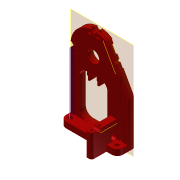
# Autodesk Inventor part: Cycl_marcoDerechoX
Saved by Autodesk Inventor 2015 SP2 (Build 190223200, 223)
## iProperties
Created: 2015-05-05
Material: Genérico
Document SubType Name: Modeling
Designer: E.Beroiz
Density: 1 g/cm^3
Appearance: Suave - Rojo
Description: Cycl_marcoDerechoX
Author: E.Beroiz
Autodesk Inventor part; units mm, degrees
ref_plane "YZ Plane" through (0, 0, 0) normal (1, 0, 0) x (0, 1, 0)
sketch "Boceto1" plane through (0, 0, 0) normal (0, 0, 1) x (1, 0, 0)
  line L0 (-49.75, 14.5) -> (49.75, 14.5)
  line L1 (49.75, 14.5) -> (49.75, -14.5)
  line L2 (49.75, -14.5) -> (-49.75, -14.5)
  line L3 (-49.75, -14.5) -> (-49.75, 14.5)
  point P0 (0, 0)
  point P1 (0, 14.5)
  point P2 (49.75, 0)
  dimension "d0" = 29
  dimension "d1" = 99.5
  constraints: 8 end point, 2 midpoint, 2 parallel, 1 horizontal, 1 horizontal alignment, 1 perpendicular, 1 vertical alignment
  measures "d0" distance of L0.end L1.end
  measures "d1" distance of L0.start L0.end
extrude "Extrusión1" add sketch "Boceto1" along normal blind 10
sketch "Boceto2" plane through (0, 0, 10) normal (0, 0, 1) x (1, 0, 0)
  line L0 (49.75, -14.5) -> (49.75, 14.5) projected
  line L1 (-49.75, 14.5) -> (49.75, 14.5)
  line L2 (49.75, 14.5) -> (49.75, 3.5)
  line L3 (49.75, 3.5) -> (-49.75, 3.5)
  line L4 (-49.75, 3.5) -> (-49.75, 14.5)
  point P0 (0, 0)
  dimension "d4" = 11
  constraints: 8 end point, 2 parallel, 1 horizontal, 1 perpendicular, 1 point on line
  measures "d4" distance of L1.end L2.end
extrude "Extrusión2" add sketch "Boceto2" along normal blind 144
sketch "Boceto3" plane through (-49.75, 3.5, 10) normal (0, -1, 0) x (1, 0, 0)
  line L0 (15, 76.5) -> (64.5, 76.5)
  line L1 (64.5, 76.5) -> (64.5, 0)
  line L2 (64.5, 0) -> (15, 0)
  line L3 (15, 0) -> (15, 76.5)
  line L4 (0, 0) -> (0, 144) projected
  point P0 (49.75, -10)
  point P1 (99.5, 0)
  dimension "d7" = 15
  dimension "d8" = 49.5
  dimension "d9" = 76.5
  constraints: 8 end point, 2 parallel, 1 horizontal, 1 horizontal alignment, 1 perpendicular
  measures "d7" distance between parallel lines of L4 L3
  measures "d8" distance of L0.start L0.end
  measures "d9" distance of L0.end L1.end
extrude "Extrusión3" cut sketch "Boceto3" against normal blind 154
fillet "Empalme1" radius 13 4 edges at (-34.75, 9, 10) (14.75, 9, 10) (-34.75, 9, 86.5) (14.75, 9, 86.5)
sketch "Boceto4" plane through (-49.75, 3.5, 154) normal (0, -1, 0) x (1, 0, 0)
  circle A0 centre (39.75, -40) radius 10.4
  line L0 (28, -67.5) -> (51.5, -67.5) projected
  point P0 (49.75, -154)
  point P1 (39.75, -67.5)
  dimension "d13" = 20.8
  dimension "d14" = 27.5
  constraints: 1 centre point, 1 midpoint, 1 vertical alignment
  measures "d13" diameter of A0
  measures "d14" distance from line of L0 A0.centre
extrude "Extrusión4" cut sketch "Boceto4" against normal through all
sketch "Boceto5" plane through (-49.75, 14.5, 0) normal (0, 1, 0) x (1, 0, 0)
  circle A0 centre (39.75, -114) radius 10.4 projected
  circle A1 centre (39.75, -114) radius 11.25
  point P0 (49.75, 0)
  dimension "d17" = 22.5
  constraints: 1 centre point, 1 coincident
  measures "d17" diameter of A1
extrude "Extrusión5" cut sketch "Boceto5" against normal blind 8
fillet "Empalme2" radius 10 2 edges at (49.75, -14.5, 5) (-49.75, -14.5, 5)
sketch "Boceto6" plane through (-49.75, 3.5, 154) normal (0, -1, 0) x (1, 0, 0)
  line L0 (0, -154) -> (99.5, -154) projected
  line L1 (69.5, -154) -> (80.5, -154)
  line L2 (80.5, -154) -> (80.5, -114)
  line L3 (80.5, -114) -> (69.5, -114)
  line L4 (69.5, -114) -> (69.5, -154)
  line L5 (64.5, -80.5) -> (64.5, -131) projected
  point P0 (49.75, -154)
  dimension "d21" = 5
  dimension "d22" = 40
  dimension "d23" = 11
  constraints: 8 end point, 2 parallel, 1 horizontal, 1 perpendicular, 1 point on line
  measures "d21" distance between parallel lines of L4 L5
  measures "d22" distance of L1.end L2.end
  measures "d23" distance of L2.end L3.end
extrude "Extrusión6" add sketch "Boceto6" along normal blind 44
fillet "Empalme3" radius 4 2 edges at (30.75, -40.5, 20) (19.75, -40.5, 20)
sketch "Boceto7" plane through (0, 0, 154) normal (0, 0, 1) x (1, 0, 0)
  line L0 (49.75, 14.5) -> (-49.75, 14.5) projected
  line L1 (-49.75, 14.5) -> (-49.75, 3.5) projected
  line L2 (-49.75, 3.5) -> (49.75, 3.5) projected
  line L3 (49.75, 3.5) -> (49.75, 14.5) projected
  line L4 (35.75, 3.5) -> (35.75, 6.5)
  arc A0 (38.75, 6.5) -> (35.75, 6.5) centre (37.25, 8.5) ccw
  line L5 (38.75, 6.5) -> (38.75, 3.5)
  point P0 (0, 0)
  dimension "d27" = 2.5
  dimension "d28" = 3
  dimension "d29" = 5
  dimension "d32" = 11
  constraints: 4 end point, 2 point on circle, 2 point on line, 1 centre point, 1 parallel, 1 perpendicular, 1 vertical
  measures "d27" radius of A0
  measures "d28" distance between parallel lines of L5 L4
  measures "d29" distance from line of L2 A0.centre
  measures "d32" distance between parallel lines of L3 L5
extrude "Extrusión7" cut sketch "Boceto7" against normal up to surface (144 mm away) contours L2 L4 A0 L5
sketch "Boceto8" plane through (19.75, 3.5, 40) normal (0, 0, 1) x (1, 0, 0)
  arc A0 (0, -40) -> (4, -44) centre (4, -40) ccw projected
  line L0 (7, -44) -> (4, -44) projected
  arc A1 (7, -44) -> (11, -40) centre (7, -40) ccw projected
  line L1 (11, 0) -> (11, -40) projected
  line L2 (0, 0) -> (11, 0) projected
  line L3 (0, 0) -> (0, -40) projected
  circle A2 centre (5.5, -38.75) radius 1.75
  circle A3 centre (5.5, -24.25) radius 1.75
  line L4 (7, -44) -> (4, -44) projected
  point P0 (-19.75, -3.5)
  point P1 (5.5, -44)
  point P2 (5.5, -44)
  dimension "d33" = 3.5
  dimension "d34" = 3.5
  dimension "d35" = 5.25
  dimension "d36" = 14.5
  constraints: 2 centre point, 2 midpoint, 2 vertical alignment
  measures "d33" diameter of A2
  measures "d34" diameter of A3
  measures "d35" distance from line of L0 A2.centre
  measures "d36" distance of A2.centre A3.centre
extrude "Extrusión8" cut sketch "Boceto8" against normal blind 14.7 contours A2 | A3
sketch "Boceto9" plane through (30.75, 3.5, 40) normal (1, 0, 0) x (0, 0, -1)
  line L0 (40, -40) -> (0, -40) projected
  line L1 (40, -18) -> (40, -40) projected
  line L2 (30, -18) -> (40, -18) projected
  line L3 (30, 0) -> (30, -18) projected
  line L4 (0, 0) -> (30, 0) projected
  line L5 (0, 0) -> (0, -40) projected
  line L6 (0, 0) -> (0, -40) projected
  arc A0 (0, -35.8) -> (0, -27.2) centre (0, -31.5) ccw
  point P0 (40, -3.5)
  point P1 (0, -44)
  dimension "d39" = 8.6
  dimension "d40" = 12.5
  constraints: 2 point on circle, 2 point on line, 1 centre point, 1 vertical alignment
  measures "d39" distance of A0.start A0.end
  measures "d40" distance of point (0, -44) A0.centre
extrude "Extrusión9" cut sketch "Boceto9" against normal through all contours L5 A0
sketch "Boceto10" plane through (30.75, 3.5, 40) normal (1, 0, 0) x (0, 0, -1)
  arc A0 (0, -35.8) -> (0, -27.2) centre (0, -31.5) ccw projected
  line L0 (0, -35.8) -> (0, -40) projected
  line L1 (40, -40) -> (0, -40) projected
  line L2 (40, -18) -> (40, -40) projected
  line L3 (30, -18) -> (40, -18) projected
  line L4 (30, 0) -> (30, -18) projected
  line L5 (0, 0) -> (30, 0) projected
  line L6 (0, 0) -> (0, -27.2) projected
  circle A1 centre (25, -5) radius 5
  line L7 (30, 0) -> (-114, 0) projected
  line L8 (30, -8) -> (30, 0) projected
  point P0 (40, -3.5)
  dimension "d43" = 10
  constraints: 2 tangent, 1 centre point
  measures "d43" diameter of A1
extrude "Extrusión10" cut sketch "Boceto10" against normal through all contours A1
sketch "Boceto11" plane through (-49.75, 14.5, 0) normal (0, 1, 0) x (1, 0, 0)
  line L0 (51.5, -86.5) -> (28, -86.5) projected
  line L1 (50.5, -86.5) -> (50.5, -81.25)
  line L2 (50.5, -81.25) -> (49.25, -80)
  line L3 (49.25, -80) -> (49.25, -74)
  line L4 (49.25, -74) -> (46.75, -74)
  line L5 (46.75, -74) -> (46.75, -80)
  line L6 (46.75, -80) -> (45.5, -81.25)
  line L7 (45.5, -81.25) -> (45.5, -86.5)
  line L8 (28, -86.5) -> (51.5, -86.5) projected
  line L9 (34, -86.5) -> (34, -81.25)
  line L10 (32.75, -80) -> (32.75, -74)
  line L11 (32.75, -74) -> (30.25, -74)
  line L12 (30.25, -74) -> (30.25, -80)
  line L13 (29, -81.25) -> (29, -86.5)
  line L14 (34, -81.25) -> (32.75, -80)
  line L15 (30.25, -80) -> (29, -81.25)
  point P0 (49.75, 0)
  point P1 (39.75, -86.5)
  dimension "d46" = 12.5
  dimension "d47" = 6
  dimension "d48" = 2.5
  dimension "d49" = 2.5
  dimension "d50" = 5
  dimension "d51" = 5
  dimension "d52" = 21.5
  dimension "d53" = 5.75
  constraints: 28 end point, 8 perpendicular, 6 horizontal alignment, 6 point on line, 2 equal length, 2 parallel, 1 midpoint, 1 vertical
  measures "d46" distance between parallel lines of L8 L11
  measures "d47" distance of L10.start L10.end
  measures "d48" distance of L10.end L11.end
  measures "d49" distance of L3.end L4.end
  measures "d50" distance between parallel lines of L13 L9
  measures "d51" distance between parallel lines of L1 L7
  measures "d52" distance between parallel lines of L13 L1
  measures "d53" distance from line of L7 point (39.75, -86.5)
extrude "Extrusión11" add sketch "Boceto11" against normal up to surface (11 mm away) contours L0 L13 L15 L12 L11 L10 L14 L9
ref_plane "Plano de trabajo1" through (-10, 3.5, 73.5) normal (1, 0, 0) x (0, 0, -1)
mirror "Simetría1" about plane through (-10, 3.5, 73.5) normal (1, 0, 0) of "Extrusión11"
sketch "Boceto12" plane through (-49.75, 3.5, 10) normal (0, -1, 0) x (1, 0, 0)
  line L0 (0, -10) -> (0, 144) projected
  arc A0 (61.5713, 137.2249) -> (0, 104) centre (39.75, 104) ccw
  line L1 (0, 0) -> (0, 144) projected
  line L2 (10, -10) -> (0, -10) projected
  circle A1 centre (39.75, 104) radius 10.4 projected
  line L3 (61.5713, 137.2249) -> (99.5, 68.75)
  line L4 (99.5, 68.75) -> (99.5, 156.8559)
  line L5 (99.5, 156.8559) -> (0, 156.8559)
  line L6 (0, 156.8559) -> (0, 104)
  line L7 (99.5, -10) -> (89.5, -10) projected
  point P0 (49.75, -10)
  dimension "d57" = 78.75
  constraints: 8 end point, 2 coincident, 2 perpendicular, 2 point on circle, 2 tangent, 1 centre point, 1 point on line, 1 vertical, 1 vertical alignment
  measures "d57" distance from line of L7 L3.end
extrude "Extrusión12" cut sketch "Boceto12" against normal through all contours L0 L6 L5 L4 L3 A0
sketch "Boceto13" plane through (0, 0, 0) normal (0, 0, -1) x (-1, 0, 0)
  line L0 (-49.75, 14.5) -> (-49.75, -4.5) projected
  line L1 (49.75, 14.5) -> (-49.75, 14.5) projected
  point P0 (0, 0)
  point P1 (-40.25, -5.5)
  point P2 (-8.75, -5.5)
  point P3 (41.25, -5.5)
  dimension "d60" = 50
  dimension "d61" = 31.5
  dimension "d62" = 9.5
  dimension "d63" = 20
  constraints: 2 horizontal alignment
  measures "d60" distance of point (41.25, -5.5) point (-8.75, -5.5)
  measures "d61" distance of point (-8.75, -5.5) point (-40.25, -5.5)
  measures "d62" distance from line of L0 point (-40.25, -5.5)
  measures "d63" distance from line of L1 point (-40.25, -5.5)
hole "Agujero1" at (40.25, -5.5, 0) at (8.75, -5.5, 0) at (-41.25, -5.5, 0) direction (0, 0, 1) diameter 3.5 end through all
sketch "Boceto16" plane through (0, 0, 10) normal (0, 0, 1) x (1, 0, 0)
  circle A0 centre (-41.25, -5.5) radius 1.75 projected
  circle A1 centre (8.75, -5.5) radius 1.75 projected
  circle A2 centre (40.25, -5.5) radius 1.75 projected
  line L0 (-39.4501, -2.3825) -> (-37.6502, -5.5)
  line L1 (-37.6502, -5.5) -> (-39.4501, -8.6175)
  line L2 (-39.4501, -8.6175) -> (-43.0499, -8.6175)
  line L3 (-43.0499, -8.6175) -> (-44.8498, -5.5)
  line L4 (-44.8498, -5.5) -> (-43.0499, -2.3825)
  line L5 (-43.0499, -2.3825) -> (-39.4501, -2.3825)
  line L6 (10.5499, -2.3825) -> (12.3498, -5.5)
  line L7 (12.3498, -5.5) -> (10.5499, -8.6175)
  line L8 (10.5499, -8.6175) -> (6.9501, -8.6175)
  line L9 (6.9501, -8.6175) -> (5.1502, -5.5)
  line L10 (5.1502, -5.5) -> (6.9501, -2.3825)
  line L11 (6.9501, -2.3825) -> (10.5499, -2.3825)
  line L12 (42.0499, -2.3825) -> (43.8498, -5.5)
  line L13 (43.8498, -5.5) -> (42.0499, -8.6175)
  line L14 (42.0499, -8.6175) -> (38.4501, -8.6175)
  line L15 (38.4501, -8.6175) -> (36.6502, -5.5)
  line L16 (36.6502, -5.5) -> (38.4501, -2.3825)
  line L17 (38.4501, -2.3825) -> (42.0499, -2.3825)
  point P0 (0, 0)
  dimension "d77" = 6.235
  constraints: 36 end point, 3 coincident, 3 horizontal, 2 horizontal alignment, 39 other
  measures "d77" distance between parallel lines of L2 L5
extrude "Extrusión15" cut sketch "Boceto16" against normal blind 2.79
ref_plane "Plano de trabajo2" through (-49.75, 9, 10) normal (0, -1, 0) x (1, 0, 0)
ref_plane "Plano de trabajo3" through (-10, 3.5, 153.75) normal (0, 0, 1) x (1, 0, 0)
sketch "Boceto17" plane through (-10, 3.5, 153.75) normal (0, 0, 1) x (1, 0, 0)
  line L0 (-39.75, 11) -> (21.8213, 11) construction
  line L1 (-39.75, 11) -> (-39.75, 0) projected
  line L2 (21.8213, 0) -> (-39.75, 0) projected
  line L3 (21.8213, 0) -> (21.8213, 11) construction
  line L4 (79.65, 5.5) -> (-59.65, 5.5) projected
  circle A0 centre (-7.25, 5.5) radius 1.875
  circle A1 centre (7.25, 5.5) radius 1.875
  line L5 (10.4, 0) -> (-10.4, 0) projected
  point P0 (10, -3.5)
  point P1 (-24.75, 0)
  point P2 (24.75, 0)
  dimension "d80" = 3.75
  dimension "d81" = 3.75
  dimension "d82" = 14.5
  dimension "d88" = 17.5
  dimension "d89" = 17.5
  constraints: 2 centre point, 2 point on line
  measures "d80" diameter of A1
  measures "d81" diameter of A0
  measures "d82" distance of A0.centre A1.centre
  measures "d88" horizontal distance of point (-24.75, 0) A0.centre
  measures "d89" horizontal distance of A1.centre point (24.75, 0)
extrude "Extrusión16" cut sketch "Boceto17" against normal blind 14.7
sketch "Boceto14" plane through (-49.75, 3.5, 10) normal (0, -1, 0) x (1, 0, 0)
  circle A0 centre (0, 104) radius 4.3
  point P0 (49.75, -10)
  dimension "d71" = 8.6
  constraints: 1 centre point
  measures "d71" diameter of A0
extrude "Extrusión13" cut sketch "Boceto14" against normal blind 20
sketch "Boceto15" plane through (-49.75, 3.5, 10) normal (0, -1, 0) x (1, 0, 0)
  arc A0 (61.5713, 137.2249) -> (0.2326, 108.2937) centre (39.75, 104) ccw projected
  circle A1 centre (39.75, 143.75) radius 4.3
  point P0 (49.75, -10)
  dimension "d74" = 8.6
  constraints: 1 centre point, 1 point on circle, 1 vertical alignment
  measures "d74" diameter of A1
extrude "Extrusión14" cut sketch "Boceto15" against normal blind 20
sketch "Boceto18" plane through (-49.75, -4.5, 0) normal (-1, 0, 0) x (0, 0, 1)
  circle A0 centre (121.2774, 13.5) radius 1.875
  circle A1 centre (106.7774, 13.5) radius 1.875
  line L0 (118.2937, 19) -> (118.2937, 8) projected
  line L1 (118.2937, 19) -> (118.2937, 8) projected
  line L2 (109.7, 19) -> (118.2937, 19) projected
  line L3 (109.7, 8) -> (109.7, 19) projected
  line L4 (118.2937, 8) -> (109.7, 8) projected
  line L5 (153.5174, 19) -> (153.5174, 8) projected
  line L6 (147.2249, 8) -> (153.5174, 8) projected
  line L7 (147.2249, 8) -> (147.2249, 19) projected
  line L8 (153.5174, 19) -> (147.2249, 19) projected
  point P0 (0, 4.5)
  point P1 (118.2937, 13.5)
  dimension "d90" = 3.75
  dimension "d91" = 3.75
  dimension "d92" = 14.5
  constraints: 2 centre point, 2 horizontal alignment, 1 midpoint, 1 other
  measures "d90" diameter of A0
  measures "d91" diameter of A1
  measures "d92" distance of A1.centre A0.centre
extrude "Extrusión17" cut sketch "Boceto18" against normal blind 14.7 contours A0 | A1
ref_plane "Plano de trabajo4" through (19.75, 3.5, 33.79) normal (0, 0, 1) x (1, 0, 0)
sketch "Boceto19" plane through (19.75, 3.5, 33.79) normal (0, 0, 1) x (1, 0, 0)
  circle A0 centre (5.5, -24.25) radius 1.75 projected
  circle A1 centre (5.5, -38.75) radius 1.75 projected
  line L0 (9.0998, -24.25) -> (7.2999, -27.3675)
  line L1 (7.2999, -27.3675) -> (3.7001, -27.3675)
  line L2 (3.7001, -21.1325) -> (7.2999, -21.1325)
  line L3 (7.2999, -21.1325) -> (9.0998, -24.25)
  line L4 (9.0998, -38.75) -> (7.2999, -41.8675)
  line L5 (7.2999, -41.8675) -> (3.7001, -41.8675)
  line L6 (3.7001, -35.6325) -> (7.2999, -35.6325)
  line L7 (7.2999, -35.6325) -> (9.0998, -38.75)
  line L8 (3.7001, -21.1325) -> (-0.5, -21.1325)
  line L9 (-0.5, -21.1325) -> (-0.5, -27.3675)
  line L10 (-0.5, -27.3675) -> (3.7001, -27.3675)
  line L11 (3.7001, -35.6325) -> (-0.5, -35.6325)
  line L12 (-0.5, -35.6325) -> (-0.5, -41.8675)
  line L13 (-0.5, -41.8675) -> (3.7001, -41.8675)
  point P0 (-19.75, -3.5)
  dimension "d96" = 6.235
  dimension "d97" = 6.235
  dimension "d98" = 6
  dimension "d99" = 6
  constraints: 28 end point, 5 horizontal, 2 coincident, 2 perpendicular, 1 vertical, 16 other
  measures "d96" distance between parallel lines of L2 L1
  measures "d97" distance between parallel lines of L5 L6
  measures "d98" distance from line of L9 A0.centre
  measures "d99" horizontal distance of L12.end A1.centre
extrude "Extrusión18" cut sketch "Boceto19" against normal blind 2.9
ref_plane "Plano de trabajo5" through (-10, 3.5, 147.54) normal (0, 0, 1) x (1, 0, 0)
sketch "Boceto20" plane through (-10, 3.5, 147.54) normal (0, 0, 1) x (1, 0, 0)
  circle A0 centre (-7.25, 5.5) radius 1.875 projected
  circle A1 centre (7.25, 5.5) radius 1.875 projected
  line L0 (-7.25, 9.0998) -> (-4.1325, 7.2999)
  line L1 (-4.1325, 7.2999) -> (-4.1325, 3.7001)
  line L2 (-10.3675, 3.7001) -> (-10.3675, 7.2999)
  line L3 (-10.3675, 7.2999) -> (-7.25, 9.0998)
  line L4 (7.25, 9.0998) -> (10.3675, 7.2999)
  line L5 (10.3675, 7.2999) -> (10.3675, 3.7001)
  line L6 (4.1325, 3.7001) -> (4.1325, 7.2999)
  line L7 (4.1325, 7.2999) -> (7.25, 9.0998)
  line L8 (-10.3675, 3.7001) -> (-10.3675, -0.5)
  line L9 (-10.3675, -0.5) -> (-4.1325, -0.5)
  line L10 (-4.1325, -0.5) -> (-4.1325, 3.7001)
  line L11 (4.1325, 3.7001) -> (4.1325, -0.5)
  line L12 (4.1325, -0.5) -> (10.3675, -0.5)
  line L13 (10.3675, -0.5) -> (10.3675, 3.7001)
  point P0 (10, -3.5)
  dimension "d103" = 6.235
  dimension "d104" = 6.235
  dimension "d105" = 6
  dimension "d106" = 6
  constraints: 28 end point, 4 perpendicular, 4 vertical, 2 coincident, 16 other
  measures "d103" distance between parallel lines of L6 L5
  measures "d104" distance between parallel lines of L1 L2
  measures "d105" distance from line of A0.centre L9
  measures "d106" distance from line of A1.centre L12
extrude "Extrusión19" cut sketch "Boceto20" against normal blind 2.8
ref_plane "Plano de trabajo6" through (-43.54, -4.5, 0) normal (-1, 0, 0) x (0, 0, 1)
sketch "Boceto22" plane through (-43.54, -4.5, 0) normal (-1, 0, 0) x (0, 0, 1)
  circle A0 centre (121.2774, 13.5) radius 1.875 projected
  line L0 (121.2774, 17.0998) -> (124.3949, 15.2999)
  line L1 (124.3949, 15.2999) -> (124.3949, 11.7001)
  line L2 (118.1599, 11.7001) -> (118.1599, 15.2999)
  line L3 (118.1599, 15.2999) -> (121.2774, 17.0998)
  circle A1 centre (106.7774, 13.5) radius 1.875 projected
  line L4 (106.7774, 17.0998) -> (109.8949, 15.2999)
  line L5 (109.8949, 15.2999) -> (109.8949, 11.7001)
  line L6 (103.6599, 11.7001) -> (103.6599, 15.2999)
  line L7 (103.6599, 15.2999) -> (106.7774, 17.0998)
  line L8 (124.3949, 11.7001) -> (124.3949, 7.5)
  line L9 (124.3949, 7.5) -> (118.1599, 7.5)
  line L10 (118.1599, 7.5) -> (118.1599, 11.7001)
  line L11 (109.8949, 11.7001) -> (109.8949, 7.5)
  line L12 (109.8949, 7.5) -> (103.6599, 7.5)
  line L13 (103.6599, 7.5) -> (103.6599, 11.7001)
  point P0 (0, 4.5)
  dimension "d111" = 6.235
  dimension "d113" = 6.235
  dimension "d114" = 6
  dimension "d115" = 6
  constraints: 28 end point, 5 vertical, 3 perpendicular, 2 coincident, 16 other
  measures "d111" distance between parallel lines of L1 L2
  measures "d113" distance between parallel lines of L6 L5
  measures "d114" distance from line of L9 A0.centre
  measures "d115" distance from line of L12 A1.centre
extrude "Extrusión20" cut sketch "Boceto22" against normal blind 2.8
sketch "Boceto25" plane through (11.8213, 3.5, 147.2249) normal (0.8747688, 0, 0.4845406) x (0.4845406, 0, -0.8747688)
  line L0 (0, 11) -> (78.2777, 11) projected
  line L1 (0, 0) -> (0, 11) projected
  line L2 (49.3844, 0) -> (0, 0) projected
  line L3 (49.3844, 3) -> (49.3844, 0) projected
  ellipse E0 centre (52.4801, 5) end of major axis (57.6396, 5) minor radius 2.5 (55.5758, 3) -> (49.3844, 3) ccw projected
  line L4 (55.5758, 0) -> (55.5758, 3) projected
  line L5 (78.2777, 0) -> (55.5758, 0) projected
  line L6 (78.2777, 11) -> (78.2777, 0) projected
  line L7 (0, 0) -> (40.5, 0)
  line L8 (40.5, 0) -> (40.5, 11)
  line L9 (40.5, 11) -> (0, 11)
  line L10 (0, 11) -> (0, 0)
  point P0 (123.0599, -3.5)
  dimension "d118" = 40.5
  constraints: 8 end point, 2 parallel, 1 horizontal, 1 perpendicular, 1 point on line, 1 other
  measures "d118" distance of L9.end L8.end
extrude "Extrusión21" cut sketch "Boceto25" against normal blind 1.5 contours L0 L8 L2 L1
sketch "Boceto26" plane through (10.5091, 3.5, 146.4981) normal (0.8747688, 0, 0.4845406) x (0.4845406, 0, -0.8747688)
  circle A0 centre (4, 3) radius 1.5 projected
  circle A1 centre (22.75, 3) radius 1.5 projected
  circle A2 centre (4, 3) radius 1.7
  circle A3 centre (22.75, 3) radius 1.7
  point P0 (123.0599, -3.5)
  dimension "d121" = 3.4
  dimension "d122" = 3.4
  constraints: 2 centre point, 2 coincident
  measures "d121" diameter of A2
  measures "d122" diameter of A3
extrude "Extrusión22" cut sketch "Boceto26" against normal blind 17 contours A0 | A1 | A2 | A3
sketch "Boceto27" plane through (10.5091, 3.5, 146.4981) normal (0.8747688, 0, 0.4845406) x (0.4845406, 0, -0.8747688)
  line L0 (0, 11) -> (40.5, 11) projected
  line L1 (6.7081, 11) -> (20.7081, 11)
  line L2 (20.7081, 11) -> (20.7081, 7)
  line L3 (20.7081, 7) -> (6.7081, 7)
  line L4 (6.7081, 7) -> (6.7081, 11)
  point P0 (123.0599, -3.5)
  dimension "d125" = 14
  dimension "d126" = 4
  constraints: 8 end point, 2 parallel, 1 horizontal, 1 perpendicular, 1 point on line
  measures "d125" distance of L2.end L3.end
  measures "d126" distance between parallel lines of L0 L3
extrude "Extrusión23" cut sketch "Boceto27" against normal blind 3
sketch "Boceto28" plane through (10.5091, 3.5, 146.4981) normal (0.8747688, 0, 0.4845406) x (0.4845406, 0, -0.8747688)
  line L0 (20.7081, 11) -> (40.5, 11) projected
  line L1 (98.954, 11) -> (2.9918, 11) projected
  line L2 (27.7081, 11) -> (31.7081, 11)
  line L3 (31.7081, 11) -> (31.7081, 2)
  line L4 (31.7081, 2) -> (27.7081, 2)
  line L5 (27.7081, 2) -> (27.7081, 11)
  line L6 (20.7081, 11) -> (20.7081, 7) projected
  point P0 (123.0599, -3.5)
  dimension "d129" = 9
  dimension "d130" = 4
  dimension "d131" = 7
  constraints: 8 end point, 2 parallel, 1 horizontal, 1 perpendicular, 1 point on line
  measures "d129" distance of L4.end L2.start
  measures "d130" distance of L3.end L4.end
  measures "d131" distance between parallel lines of L5 L6
extrude "Extrusión24" cut sketch "Boceto28" against normal blind 3
chamfer "Chaflán1" distance 0.8 angle 30 1 edges at (-21.25, 14.5, 114) measured on face at (1.1043, 9.1667, 115.8046)
ref_plane "Plano de trabajo7" through (8.2347, 3.5, 145.2383) normal (0.8747688, 0, 0.4845406) x (0.4845406, 0, -0.8747688)
sketch "Boceto30" plane through (8.2347, 3.5, 145.2383) normal (0.8747688, 0, 0.4845406) x (0.4845406, 0, -0.8747688)
  circle A0 centre (4, 3) radius 2 projected
  circle A1 centre (22.75, 3) radius 1.5 projected
  line L0 (4, 6.5998) -> (7.1175, 4.7999)
  line L1 (7.1175, 4.7999) -> (7.1175, 1.2001)
  line L2 (0.8825, 1.2001) -> (0.8825, 4.7999)
  line L3 (0.8825, 4.7999) -> (4, 6.5998)
  line L4 (22.75, 6.5998) -> (25.8675, 4.7999)
  line L5 (25.8675, 4.7999) -> (25.8675, 1.2001)
  line L6 (19.6325, 1.2001) -> (19.6325, 4.7999)
  line L7 (19.6325, 4.7999) -> (22.75, 6.5998)
  line L8 (0.8825, 1.2001) -> (0.8825, -0.7999)
  line L9 (0.8825, -0.7999) -> (7.1175, -0.7999)
  line L10 (7.1175, -0.7999) -> (7.1175, 1.2001)
  line L11 (19.6325, 1.2001) -> (19.6325, -0.7999)
  line L12 (19.6325, -0.7999) -> (25.8675, -0.7999)
  line L13 (25.8675, -0.7999) -> (25.8675, 1.2001)
  point P0 (123.0599, -3.5)
  dimension "d138" = 6.235
  dimension "d139" = 6.235
  dimension "d140" = 2
  dimension "d141" = 2
  constraints: 28 end point, 5 vertical, 3 perpendicular, 2 coincident, 16 other
  measures "d138" distance between parallel lines of L1 L2
  measures "d139" distance between parallel lines of L5 L6
  measures "d140" distance of L2.start L8.end
  measures "d141" distance of L6.start L11.end
extrude "Extrusión25" cut sketch "Boceto30" against normal blind 2.8 contours A0 | A1 | L0 L1 L10 L9 L8 L2 L3 | L4 L5 L13 L12 L11 L6 L7
fillet "Empalme4" radius 0.5 4 edges at (-49.75, 9, 109.7) (-49.5174, 9, 118.2937) (-5.7063, 9, 153.5174) (-14.2937, 9, 153.5174)
fillet "Empalme5" radius 0.5 2 edges at (25.25, -23.7, 40) (25.25, -32.3, 40)
